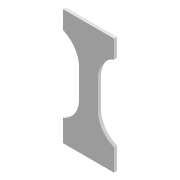
# Autodesk Inventor part: dogbone
Saved by Autodesk Inventor 2021 (Build 250183000, 183)
## iProperties
Created: 2021-07-02
Part Number: dogbone
Material: Speckle pattern
Document SubType Name: Modeling
Designer: mcgheealex
Density: 1 g/cm^3
Appearance: Default
Author: mcgheealex
Autodesk Inventor part; units mm, degrees
ref_plane "YZ Plane" through (0, 0, 0) normal (1, 0, 0) x (0, 1, 0)
ref_plane "XZ Plane" through (0, 0, 0) normal (0, 1, 0) x (-1, 0, 0)
ref_plane "XY Plane" through (0, 0, 0) normal (0, 0, 1) x (1, 0, 0)
sketch "Sketch1" plane through (0, 0, 0) normal (0, 0, 1) x (1, 0, 0)
  line L0 (-31.9674, 70.0993) -> (31.9674, 70.0993)
  line L1 (31.9674, 70.0993) -> (31.9674, -74.8548)
  line L2 (31.9674, -74.8548) -> (-31.9674, -74.8548)
  line L3 (-31.9674, -74.8548) -> (-31.9674, 70.0993)
  circle A0 centre (-44.1203, 17.5249) radius 32.3435
  circle A1 centre (44.1203, 17.5249) radius 32.3435
  line L4 (0, 0) -> (0, 29.7658) construction
  line L5 (-44.1203, 17.5249) -> (44.1203, 17.5249)
  line L6 (44.1203, 17.5249) -> (44.1203, -17.5249)
  line L7 (44.1203, -17.5249) -> (-44.1203, -17.5249)
  line L8 (-44.1203, -17.5249) -> (-44.1203, 17.5249)
  line L9 (0, 0) -> (9.4229, 0) construction
  circle A2 centre (44.1203, -17.5249) radius 32.3435
  circle A3 centre (-44.1203, -17.5249) radius 32.3435
  line L10 (-11.7768, 40.2762) -> (11.7768, 40.2762)
  line L11 (11.7768, 40.2762) -> (11.7768, -36.31)
  line L12 (11.7768, -36.31) -> (-11.7768, -36.31)
  line L13 (-11.7768, -36.31) -> (-11.7768, 40.2762)
  point P0 (-31.9674, 47.4983)
  point P1 (-11.7768, 17.5249)
  point P2 (-11.7768, -17.5249)
  point P3 (-31.9674, -47.4983)
  point P4 (31.9674, -47.4983)
  point P5 (11.7768, -17.5249)
  point P6 (11.7768, 17.5249)
  point P7 (31.9674, 47.4983)
  constraints: 28 end point, 6 parallel, 4 centre point, 4 horizontal, 4 tangent, 3 perpendicular, 2 coincident, 2 equal radius, 1 symmetric about line, 1 vertical, 2 other
extrude "Extrusion1" add sketch "Sketch1" along normal blind 3.81 contours L0 L1 A1 L11 L10 L13 A0 L3 | L13 L10 L11 L5 | L5 L11 L7 L13 | L13 L12 L11 A2 L1 L2 L3 A3 | L7 L11 L12 L13
sketch "Sketch2" plane through (0, 0, 3.81) normal (0, 0, 1) x (1, 0, 0)
  line L0 (-20.9663, 30.173) -> (25.2183, 30.173)
  line L1 (25.2183, 30.173) -> (25.2183, -34.1474)
  line L2 (25.2183, -34.1474) -> (-20.9663, -34.1474)
  line L3 (-20.9663, -34.1474) -> (-20.9663, 30.173)
  point P0 (0, 0)
  constraints: 8 end point, 2 parallel, 1 horizontal, 1 perpendicular
extrude "Extrusion2" cut sketch "Sketch2" against normal blind 0.0025
body "Solid1"
